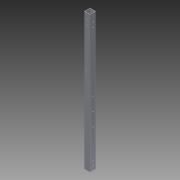
# Autodesk Inventor part: Rebuild Edge Mount 1
Saved by Autodesk Inventor 2014 SP1 (Build 180222100, 222)
## iProperties
Created: 2013-01-21
Part Number: Rebuild Edge Mount 1
Material: Aluminum 6061
Document SubType Name: Modeling
Designer: actoennies
Density: 2.71 g/cm^3
Mass: 241.272 g
Surface Area: 1132 cm^2
Volume: 89.0301 cm^3
Appearance: Aluminum - Flat
Author: actoennies
Autodesk Inventor part; units mm, degrees
ref_plane "YZ Plane" through (0, 0, 0) normal (1, 0, 0) x (0, 1, 0)
ref_plane "XZ Plane" through (0, 0, 0) normal (0, 1, 0) x (-1, 0, 0)
ref_plane "XY Plane" through (0, 0, 0) normal (0, 0, 1) x (1, 0, 0)
sketch "Sketch1" plane through (0, 0, 0) normal (0, 1, 0) x (-1, 0, 0)
  line L0 (0, 0) -> (-25.4, 0)
  line L1 (-25.4, 0) -> (-25.4, 25.4)
  line L2 (-25.4, 25.4) -> (0, 25.4)
  line L3 (0, 25.4) -> (0, 0)
  line L4 (-1.5875, 23.8125) -> (-23.8125, 23.8125)
  line L5 (-23.8125, 23.8125) -> (-23.8125, 1.5875)
  line L6 (-23.8125, 1.5875) -> (-1.5875, 1.5875)
  line L7 (-1.5875, 1.5875) -> (-1.5875, 23.8125)
  dimension "d0" = 25.4
  dimension "d2" = 25.4
  dimension "d3" = 1.5875
  constraints: 16 end point, 4 parallel, 2 perpendicular, 1 horizontal, 3 other
  measures "d0" distance of L0.end L1.end
  measures "d2" distance of L1.end L2.end
  measures "d3" distance between parallel lines of L2 L4
extrude "Extrusion1" add sketch "Sketch1" along normal blind 596.9
sketch "Sketch7" plane through (25.4, 0, 0) normal (0, 0, -1) x (-1, 0, 0)
  circle A0 centre (12.7, 552.45) radius 3.3782
  circle A1 centre (12.7, 574.675) radius 3.3782
  constraints: 2 centre point, 4 other
extrude "Extrusion6" cut sketch "Sketch7" against normal blind 25.4
sketch "Sketch8" plane through (25.4, 0, 25.4) normal (1, 0, 0) x (0, 0, -1)
  circle A0 centre (12.7, 565.15) radius 3.3782
  circle A1 centre (12.7, 542.925) radius 3.3782
  circle A2 centre (12.7, 19.05) radius 3.302 projected
  circle A3 centre (12.7, 38.1) radius 3.302 projected
  arc A4 (25.4, 47.625) -> (22.225, 50.8) centre (22.225, 47.625) ccw projected
  line L0 (22.225, 50.8) -> (3.175, 50.8) projected
  arc A5 (3.175, 50.8) -> (0, 47.625) centre (3.175, 47.625) ccw projected
  line L1 (0, 47.625) -> (0, 4.445) projected
  line L2 (0, 4.445) -> (25.4, 4.445) projected
  line L3 (25.4, 47.625) -> (25.4, 4.445) projected
  arc A6 (22.225, 155.2575) -> (25.4, 158.4325) centre (22.225, 158.4325) ccw projected
  line L4 (3.175, 155.2575) -> (22.225, 155.2575) projected
  arc A7 (0, 158.4325) -> (3.175, 155.2575) centre (3.175, 158.4325) ccw projected
  line L5 (0, 177.4825) -> (0, 158.4325) projected
  arc A8 (0, 177.4825) -> (-3.175, 180.6575) centre (-3.175, 177.4825) ccw projected
  line L6 (-7.0866, 180.6575) -> (-3.175, 180.6575) projected
  line L7 (-7.0866, 180.6575) -> (-7.0866, 244.1575) projected
  line L8 (-3.175, 244.1575) -> (-7.0866, 244.1575) projected
  arc A9 (-3.175, 244.1575) -> (0, 247.3325) centre (-3.175, 247.3325) ccw projected
  line L9 (0, 291.7825) -> (0, 247.3325) projected
  arc A10 (3.175, 294.9575) -> (0, 291.7825) centre (3.175, 291.7825) ccw projected
  line L10 (22.225, 294.9575) -> (3.175, 294.9575) projected
  arc A11 (25.4, 291.7825) -> (22.225, 294.9575) centre (22.225, 291.7825) ccw projected
  line L11 (25.4, 158.4325) -> (25.4, 291.7825) projected
  circle A12 centre (12.7, 166.0525) radius 3.302 projected
  circle A13 centre (12.7, 199.7075) radius 3.302 projected
  circle A14 centre (12.7, 225.1075) radius 3.302 projected
  circle A15 centre (12.7, 253.6825) radius 3.302 projected
  circle A16 centre (12.7, 282.2575) radius 3.302 projected
  constraints: 2 centre point, 4 other
extrude "Extrusion7" cut sketch "Sketch8" against normal blind 25.4 contours A0 | A1 | A2 | A3 | A12 | A14 | A16
sketch "Sketch9" plane through (25.4, 0, 0) normal (0, 0, -1) x (-1, 0, 0)
  circle A0 centre (12.7, 431.8) radius 3.3782 projected
  line L0 (25.4, 440.055) -> (0, 440.055) projected
  line L1 (0, 368.3) -> (0, 440.055) projected
  line L2 (25.4, 368.3) -> (0, 368.3) projected
  line L3 (25.4, 440.055) -> (25.4, 368.3) projected
  circle A1 centre (12.7, 431.8) radius 3.3782 projected
  circle A2 centre (12.7, 381) radius 3.3782 projected
extrude "Extrusion8" cut sketch "Sketch9" against normal blind 25.4 contours A0 | A2
body "Solid1"
